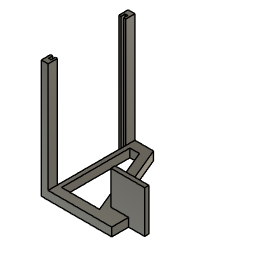
KobraNeoCameraPlatform (Autodesk Fusion 360 design; units mm, degrees)
Autodesk Fusion 360 part; units mm, degrees
note: some values were not read from the file. Set by a fixed rule: which sketch regions a step uses.
sketch "Sketch1" plane through (0, 0, 0) normal (1, 0, 0) x (0, 1, 0)
  line L0 (0, 0) -> (11, 0)
  line L1 (11, 8) -> (0, 8)
  line L2 (0, 8) -> (0, 0)
  line L3 (11, 5.5) -> (6, 5.5)
  line L4 (6, 5.5) -> (6, 2.5)
  line L5 (6, 2.5) -> (11, 2.5)
  line L6 (11, 0) -> (11, 2.5)
  line L7 (11, 5.5) -> (11, 8)
  line L8 (92, 0) -> (92, 2.5012)
  line L9 (97, 5.5) -> (97, 2.5)
  line L10 (103, 0) -> (92, 0)
  line L11 (92, 5.5) -> (92, 8)
  line L12 (92, 5.5) -> (97, 5.5)
  line L13 (92, 8) -> (103, 8)
  line L14 (97, 2.5) -> (92, 2.5012)
  line L15 (103, 8) -> (103, 0)
  dimension "d1" = 11
  dimension "d2" = 8
  dimension "d5" = 3
  dimension "d6" = 5
  dimension "d7" = 2.5
  dimension "d11" = 11
  dimension "d12" = 8
  dimension "d13" = 3
  dimension "d15" = 2.5
  dimension "d16" = 91
  dimension "d39" = 5
  constraint horizontal L0
  constraint vertical L6
  constraint horizontal L1
  constraint vertical L2
  constraint coincident L0.start L2.end
  constraint horizontal L3
  constraint vertical L4
  constraint horizontal L5
  constraint coincident L3.start L6
  constraint collinear L6 L7
  constraint coincident L11.start L8
  constraint collinear L8 L11
  constraint parallel L7 L11
  constraint collinear L0 L10
  constraint perpendicular L10 L15
  constraint parallel L10 L13
  constraint equal L12 L14
  measures "d1" distance of L0.start L0.end
  measures "d2" distance of L0.start L1.end
  measures "d5" distance of L3.end L4.end
  measures "d6" distance of L3.start L3.end
  measures "d7" distance of L1 L3
  measures "d11" distance of L8.start L10.start
  measures "d12" distance of L13.end L10.start
  measures "d13" distance of L9.start L9.end
  measures "d15" distance of L12 L13
  measures "d16" distance of L4 L9
  measures "d39" distance of L9 L11
extrude "Extrude1" add sketch "Sketch1" along normal blind 140 makes body 1 at (46.6667, 7.3333, 8) makes body 2 at (46.6667, 95.6667, 8)
sketch "Sketch2" plane through (140, 0, 0) normal (1, 0, 0) x (0, 1, 0)
  line L0 (6, 5.5) -> (11, 5.5)
  line L1 (11, 5.5) -> (11, 8)
  line L2 (11, 8) -> (0, 8)
  line L3 (0, 8) -> (0, 0)
  line L4 (0, 0) -> (11, 0)
  line L5 (11, 0) -> (11, 2.5)
  line L6 (11, 2.5) -> (6, 2.5)
  line L7 (6, 2.5) -> (6, 5.5)
  line L8 (0, 8) -> (10.1021, 8)
  line L9 (11, 13) -> (11, 58)
  line L10 (103, 8) -> (92, 8)
  line L11 (92, 8) -> (103, 8)
  line L12 (11, 58) -> (0, 58)
  line L13 (11, 58) -> (92, 24.342)
  line L14 (10.1021, 8) -> (92, 8)
  line L15 (92, 13) -> (11, 13)
  line L16 (92, 24.342) -> (92, 13)
  line L17 (92, 8) -> (92, 8)
  line L18 (25, 83.488) -> (25, 62.5795)
  line L19 (103, 8) -> (103, 30.0279)
  line L20 (25, 62.5795) -> (103, 30.0279)
  line L21 (103, 0) -> (103, 8)
  line L22 (0, 83.488) -> (25, 83.488)
  line L23 (0, 83.488) -> (0, 8)
  point P0 (92, 8)
  dimension "d40" = 5
  dimension "d41" = 50
  dimension "d42" = 11
  dimension "d43" = 25
  dimension "d44" = 11
  constraint horizontal L8
  constraint vertical L9
  constraint coincident L2.end L3.start
  constraint horizontal L11
  constraint vertical L16
  constraint coincident P0 L10.end
  constraint horizontal L12
  constraint equal L4 L12
  constraint horizontal L14
  constraint horizontal L15
  constraint collinear L16 L17
  constraint vertical L18
  constraint perpendicular L11 L19
  constraint collinear L19 L21
  constraint perpendicular L18 L22
  constraint perpendicular L8 L23
  measures "d40" distance of L14 L15
  measures "d41" distance of L1.end L9.end
  measures "d42" distance of L16 L19
  measures "d43" distance of L22.start L18.start
  measures "d44" distance of L9 L23
extrude "Extrude2" add sketch "Sketch2" against normal blind 10 contours L2 L8 L10 L11 L14 L18 L19 L20 L22 L23 bodies 1 2
sketch "Sketch4" plane through (0, 25, 0) normal (0, 1, 0) x (-1, 0, 0)
  line L0 (-140, 83.488) -> (-140, 62.5795)
  line L1 (-130, 62.5795) -> (-130, 83.488)
  line L2 (-140, 62.5795) -> (-90, 62.5795)
  line L3 (-90, 62.5795) -> (-90, 102.5795)
  line L4 (-90, 102.5795) -> (-140, 102.5795)
  line L5 (-140, 102.5795) -> (-140, 62.5795)
  line L6 (-140, 62.5795) -> (-130, 62.5795)
  line L7 (-130, 83.488) -> (-140, 83.488)
  dimension "d35" = 50
  dimension "d36" = 40
  constraint horizontal L2
  constraint vertical L3
  constraint horizontal L4
  constraint vertical L5
  constraint coincident L0.end L2.start
  measures "d35" distance of L0.end L2.end
  measures "d36" distance of L0.end L4.end
extrude "Extrude4" add sketch "Sketch4" against normal blind 5 bodies 1
move_body "Move1" bodies 1 to x (0, 0, -1) y (0, 1, 0) z (1, 0, 0) at (-44, -30, 140)
